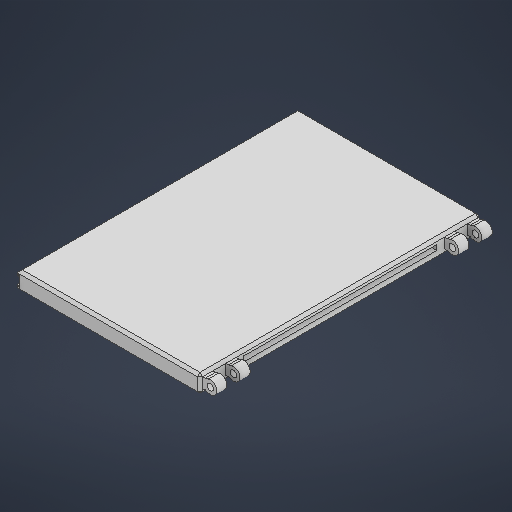
# Autodesk Inventor part: Деталь1
Saved by Autodesk Inventor 2025.1 (Build 291241000, 241)
## iProperties
Created: 2025-05-09
Part Number: Деталь1
Material: Типовые
Document SubType Name: Modeling
Designer: bogda
Density: 1 g/cm^3
Appearance: По умолчанию
Author: bogda
Autodesk Inventor part; units mm, degrees
ref_plane "YZ Plane" through (0, 0, 0) normal (1, 0, 0) x (0, 1, 0)
ref_plane "XZ Plane" through (0, 0, 0) normal (0, 1, 0) x (-1, 0, 0)
ref_plane "XY Plane" through (0, 0, 0) normal (0, 0, 1) x (1, 0, 0)
sketch "Эскиз1" plane through (0, 0, 0) normal (0, 1, 0) x (-1, 0, 0)
  line L0 (33.5, 52.5) -> (-33.5, 52.5)
  line L1 (-33.5, 52.5) -> (-33.5, -52.5)
  line L2 (-33.5, -52.5) -> (33.5, -52.5)
  line L3 (33.5, -52.5) -> (33.5, 52.5)
  line L4 (33.5, 52.5) -> (-33.5, -52.5) construction
  line L5 (-33.5, 52.5) -> (33.5, -52.5) construction
  line L6 (35.5, 54.5) -> (-35.5, 54.5)
  line L7 (-35.5, 54.5) -> (-35.5, -54.5)
  line L8 (-35.5, -54.5) -> (35.5, -54.5)
  line L9 (35.5, -54.5) -> (35.5, 54.5)
  point P0 (0, 0)
  dimension "d0" = 67
  dimension "d1" = 105
  dimension "d2" = 2
  constraints: 20 end point, 4 parallel, 2 midpoint, 2 perpendicular, 1 horizontal, 3 other
  measures "d0" distance of L2.end L1.end
  measures "d1" distance of L1.end L0.end
  measures "d2" distance between parallel lines of L3 L9
extrude "Выдавливание1" add sketch "Эскиз1" against normal blind 2 contours L3 L2 L1 L0 | L9 L8 L7 L6
extrude "Выдавливание2" add sketch "Эскиз1" against normal blind 6
sketch "Эскиз2" plane through (0, -6, 0) normal (0, -1, 0) x (1, 0, 0)
  line L0 (-33.5, -52.5) -> (-33.5, 52.5) projected
  line L1 (-33.5, -52.5) -> (-33.5, -49.5)
  line L2 (-33.5, -49.5) -> (33.5, -49.5)
  line L3 (33.5, 52.5) -> (33.5, -52.5) projected
  line L4 (33.5, -49.5) -> (26.5, -49.5)
  line L5 (26.5, -49.5) -> (26.5, 52.5)
  line L6 (-33.5, 52.5) -> (33.5, 52.5) projected
  line L7 (26.5, 52.5) -> (26.5, 49.5)
  line L8 (26.5, 49.5) -> (-33.5, 49.5)
  line L9 (-33.5, 49.5) -> (-30.5, 49.5)
  line L10 (-30.5, 49.5) -> (-30.5, -49.5)
  line L11 (33.5, -52.5) -> (-33.5, -52.5) projected
  line L12 (-33.5, -52.5) -> (33.5, -52.5)
  point P0 (0, 0)
  dimension "d7" = 3
  dimension "d8" = 7
  dimension "d9" = 3
  dimension "d10" = 3
  constraints: 18 end point, 8 point on line, 5 perpendicular
  measures "d7" distance of L0.start L1.end
  measures "d8" distance of L2.end L4.end
  measures "d9" distance of L5.end L7.end
  measures "d10" distance of L8.end L9.end
extrude "Выдавливание3" add sketch "Эскиз2" against normal blind 1 contours L0 L2 L3 L11 | L0 L8 L10 L2 | L0 L6 L5 L8 | L2 L5 L6 L3
sketch "Эскиз3" plane through (35.5, 0, 54.5) normal (1, 0, 0) x (0, 0, -1)
  line L0 (109, 0) -> (109, -6) projected
  line L1 (109, 0) -> (92, 0)
  line L2 (0, 0) -> (109, 0) projected
  line L3 (92, 0) -> (92, -2)
  line L4 (2, -5) -> (107, -5) projected
  line L5 (92, -2) -> (17, -2)
  line L6 (0, 0) -> (0, -6) projected
  line L7 (17, -2) -> (17, -4)
  line L8 (17, -4) -> (92, -4)
  line L9 (92, -4) -> (92, -2)
  line L10 (109, 0) -> (94, 0)
  line L11 (94, 0) -> (94, -6)
  line L12 (94, -6) -> (109, -6)
  line L13 (109, 0) -> (109, -6)
  line L14 (108, -5) -> (95, -5)
  line L15 (95, -5) -> (95, -1)
  line L16 (95, -1) -> (108, -1)
  line L17 (108, -1) -> (108, -5)
  line L18 (0, 0) -> (15, 0)
  line L19 (15, 0) -> (15, -6)
  line L20 (104, -6) -> (5, -6) projected
  line L21 (0, -6) -> (109, -6) projected
  line L22 (0, -6) -> (15, -6)
  line L23 (0, -6) -> (0, 0)
  line L24 (14, -5) -> (14, -1)
  line L25 (14, -1) -> (1, -1)
  line L26 (1, -1) -> (1, -5)
  line L27 (1, -5) -> (14, -5)
  line L28 (108, -5) -> (104, -5)
  line L29 (104, -5) -> (104, -1)
  line L30 (95, -5) -> (99, -5)
  line L31 (99, -5) -> (99, -1)
  line L32 (1, -5) -> (5, -5)
  line L33 (5, -5) -> (5, -1)
  line L34 (14, -5) -> (10, -5)
  line L35 (10, -5) -> (10, -1)
  point P0 (54.5, 0)
  point P1 (5, -5)
  point P2 (10, -5)
  point P3 (14, -5)
  dimension "d13" = 17
  dimension "d14" = 2
  dimension "d15" = 75
  dimension "d16" = 2
  dimension "d17" = 15
  dimension "d18" = 1
  dimension "d19" = 15
  dimension "d20" = 1
  dimension "d21" = 4
  dimension "d22" = 4
  dimension "d23" = 4
  dimension "d24" = 4
  constraints: 60 end point, 16 perpendicular, 12 point on line, 2 collinear, 6 other
  measures "d13" distance of L0.start L1.end
  measures "d14" distance of L1.end L3.end
  measures "d15" distance of L3.end L5.end
  measures "d16" distance of L5.end L7.end
  measures "d17" distance of L0.start L10.end
  measures "d18" distance between parallel lines of L12 L14
  measures "d19" distance of L2.start L18.end
  measures "d20" distance between parallel lines of L22 L27
  measures "d21" distance of L14.start L28.end
  measures "d22" distance of L14.end L30.end
  measures "d23" distance of L26.end L32.end
  measures "d24" distance of L24.start L34.end
extrude "Выдавливание4" cut sketch "Эскиз3" against normal blind 3 contours L9 L8 L7 L5
extrude "Выдавливание5" add sketch "Эскиз3" along normal blind 1 contours L27 L26 L25 L33 L4 | L35 L25 L24 L4 | L15 L16 L31 L4 | L29 L16 L17 L14 L4
sketch "Эскиз4" plane through (35.5, -5, -53.5) normal (0, 0, -1) x (-1, 0, 0)
  line L0 (-1, 4) -> (-1, 0) projected
  line L1 (-1, 0) -> (-1, 2)
  line L2 (-1, 2) -> (-3, 2)
  circle A0 centre (-3, 2) radius 2.5
  line L3 (-1, 0) -> (-2.2643, -0.3893)
  line L4 (-1, 4) -> (-2.2643, 4.3893)
  circle A1 centre (-3, 2) radius 1.25
  point P0 (35.5, 5)
  dimension "d29" = 2
  dimension "d30" = 2
  dimension "d31" = 5
  dimension "d32" = 2.5
  constraints: 8 end point, 2 centre point, 2 coincident, 2 point on circle, 2 tangent, 1 midpoint, 1 perpendicular
  measures "d29" distance of L0.end L1.end
  measures "d30" distance of L1.end L2.end
  measures "d31" diameter of A0
  measures "d32" diameter of A1
extrude "Выдавливание6" add sketch "Эскиз4" against normal blind 107 contours L0 A0 L4 | L0 A0 | A0 L0 L3 picked at (-1.2977, 1.3064)
sketch "Эскиз5" plane through (35.5, -5, -49.5) normal (0, 0, 1) x (1, 0, 0)
  line L0 (1, 0) -> (1, 4) projected
  line L1 (1, 0) -> (1, -1.4659)
  line L2 (1, -1.4659) -> (6.5669, -1.4659)
  line L3 (6.5669, -1.4659) -> (6.5669, 5)
  line L4 (6.5669, 5) -> (1, 5)
  line L5 (1, 5) -> (1, 4)
  line L6 (1, 4) -> (1, 0)
  point P0 (-35.5, 5)
  constraints: 12 end point, 4 perpendicular, 1 collinear, 1 point on line, 1 vertical
extrude "Выдавливание7" cut sketch "Эскиз5" along normal blind 5
sketch "Эскиз6" plane through (35.5, -5, -40.5) normal (0, 0, 1) x (1, 0, 0)
  line L0 (1, 0) -> (1, 4) projected
  line L1 (1, 0) -> (1, -1.1885)
  line L2 (1, -1.1885) -> (6.8207, -1.1885)
  line L3 (6.8207, -1.1885) -> (6.8207, 5)
  line L4 (6.8207, 5) -> (1, 5)
  line L5 (1, 5) -> (1, 4)
  line L6 (1, 4) -> (1, 0)
  point P0 (-35.5, 5)
  constraints: 12 end point, 4 perpendicular, 1 collinear, 1 point on line, 1 vertical
extrude "Выдавливание8" cut sketch "Эскиз6" along normal blind 81
sketch "Эскиз7" plane through (35.5, -5, 44.5) normal (0, 0, 1) x (1, 0, 0)
  line L0 (1, 0) -> (1, 4) projected
  line L1 (1, 4) -> (1, 5.6826)
  line L2 (1, 5.6826) -> (6.1559, 5.6826)
  line L3 (6.1559, 5.6826) -> (6.1559, -0.9821)
  line L4 (6.1559, -0.9821) -> (1, -0.9821)
  line L5 (1, -0.9821) -> (1, 0)
  line L6 (1, 0) -> (1, 4)
  point P0 (-35.5, 5)
  constraints: 12 end point, 3 perpendicular, 2 collinear, 1 point on line, 1 vertical
extrude "Выдавливание9" cut sketch "Эскиз7" along normal blind 5
sketch "Эскиз8" plane through (-35.5, 0, -54.5) normal (-1, 0, 0) x (0, 0, 1)
  line L0 (1, -5) -> (5, -5) projected
  line L1 (5, -1) -> (1, -1) projected
  line L2 (0, 0) -> (0, -6) projected
  line L3 (0, -5) -> (2, -5)
  line L4 (2, -5) -> (2, -2)
  line L5 (0, 0) -> (109, 0) projected
  line L6 (107, -2) -> (107, -5) projected
  line L7 (2, -2) -> (107, -2)
  line L8 (107, -2) -> (107, -5)
  line L9 (107, -5) -> (2, -5)
  point P0 (54.5, 0)
  dimension "d41" = 2
  dimension "d42" = 3
  constraints: 10 end point, 2 collinear, 2 point on line, 1 perpendicular
  measures "d41" distance of L3.start L3.end
  measures "d42" distance of L3.end L4.end
extrude "Выдавливание10" cut sketch "Эскиз8" against normal blind 5
sketch "Эскиз9" plane through (-35.5, 0, 54.5) normal (0, 0, 1) x (1, 0, 0)
  line L0 (0, 0) -> (0, -2)
  line L1 (0, 0) -> (0, -6) projected
  line L2 (0, -2) -> (0.5, -2)
  line L3 (0.5, -2) -> (0.5, 0)
  line L4 (0.5, 0) -> (1, 0)
  line L5 (1, 0) -> (1, -5)
  line L6 (1, -5) -> (1, -5.5)
  line L7 (1, -5.5) -> (0.5, -5.5)
  line L8 (0.5, -5.5) -> (0.5, -5)
  line L9 (0.5, -5) -> (0, -5)
  line L10 (0, -5) -> (0, -2)
  line L11 (0.5, 0) -> (0.5, -1)
  line L12 (0.5, -1) -> (1, -1)
  point P0 (35.5, 0)
  dimension "d45" = 2
  dimension "d46" = 0.5
  dimension "d47" = 0.5
  dimension "d48" = 5
  dimension "d49" = 0.5
  dimension "d50" = 1
  constraints: 24 end point, 8 perpendicular, 6 point on line, 1 midpoint
  measures "d45" distance of L0.start L0.end
  measures "d46" distance of L0.end L2.end
  measures "d47" distance of L3.end L4.end
  measures "d48" distance of L4.end L5.end
  measures "d49" distance of L5.end L6.end
  measures "d50" distance of L3.end L11.end
extrude "Выдавливание11" cut sketch "Эскиз9" against normal blind 110 contours L2 L3 L12 L5 L6 L7 L8 L9 L1
sketch "Эскиз10" plane through (0, -6, 0) normal (0, -1, 0) x (1, 0, 0)
  line L0 (35.5, 54.5) -> (-35.5, 54.5) projected
  line L1 (-35.5, 54.5) -> (-35.5, 52.5)
  line L2 (-35.5, 52.5) -> (35.5, 52.5)
  line L3 (35.5, -54.5) -> (35.5, 54.5) projected
  line L4 (35.5, 52.5) -> (33.5, 52.5)
  line L5 (33.5, 52.5) -> (33.5, -54.5)
  line L6 (-35.5, -54.5) -> (35.5, -54.5) projected
  line L7 (33.5, -54.5) -> (33.5, -52.5)
  line L8 (33.5, -52.5) -> (-35.5, -52.5)
  line L9 (-35.5, -52.5) -> (-33.5, -52.5)
  line L10 (-33.5, -52.5) -> (-33.5, 52.5)
  line L11 (-35.5, 52.5) -> (-35.5, -52.5)
  line L12 (-35.5, -52.5) -> (-35.5, -54.5)
  line L13 (28.1404, -7.8899) -> (28.1404, 8.4295) construction
  line L14 (28.1404, 8.4295) -> (34.5634, 8.4295) construction
  line L15 (34.5634, 8.4295) -> (34.5634, -7.8899) construction
  line L16 (34.5634, -7.8899) -> (28.1404, -7.8899) construction
  spline S0 degree 2 poles (29.8027, -5.1778) (30.2201, -5.1778) (30.892, -5.5162) (31.0797, -5.8002) knots 0 0 0 1 2 2 2
  spline S1 degree 2 poles (31.0797, -5.8002) (31.2254, -6.0324) (31.3242, -6.5091) (31.3242, -6.8796) knots 0 0 0 1 2 2 2
  line L17 (31.3242, -6.8796) -> (31.3242, -7.5811)
  line L18 (31.3242, -7.5811) -> (28.2762, -7.5811)
  line L19 (28.2762, -7.5811) -> (28.2762, -6.887)
  spline S2 degree 2 poles (28.2762, -6.887) (28.2762, -6.4573) (28.4047, -5.9682) (28.5183, -5.7953) knots 0 0 0 1 2 2 2
  spline S3 degree 2 poles (28.5183, -5.7953) (28.7134, -5.5014) (29.3581, -5.1778) (29.8027, -5.1778) knots 0 0 0 1 2 2 2
  spline S4 degree 2 poles (29.7978, -5.6002) (29.447, -5.6002) (28.9506, -5.8323) (28.8098, -6.0621) knots 0 0 0 1 2 2 2
  spline S5 degree 2 poles (28.8098, -6.0621) (28.7134, -6.2251) (28.627, -6.5931) (28.627, -6.8673) knots 0 0 0 1 2 2 2
  line L20 (28.627, -6.8673) -> (28.627, -7.176)
  line L21 (28.627, -7.176) -> (30.9735, -7.176)
  line L22 (30.9735, -7.176) -> (30.9735, -6.8673)
  spline S6 degree 2 poles (30.9735, -6.8673) (30.9735, -6.5981) (30.887, -6.1905) (30.771, -6.025) knots 0 0 0 1 2 2 2
  spline S7 degree 2 poles (30.771, -6.025) (30.6277, -5.8126) (30.1535, -5.6002) (29.7978, -5.6002) knots 0 0 0 1 2 2 2
  line L23 (31.3242, -2.9894) -> (31.3242, -3.3747)
  line L24 (31.3242, -3.3747) -> (31.0723, -3.3747)
  spline S8 degree 2 poles (31.0723, -3.3747) (31.2279, -3.5525) (31.3885, -3.8712) (31.3885, -4.0688) knots 0 0 0 1 2 2 2
  spline S9 degree 2 poles (31.3885, -4.0688) (31.3885, -4.217) (31.2897, -4.4812) (31.1835, -4.5776) knots 0 0 0 1 2 2 2
  spline S10 degree 2 poles (31.1835, -4.5776) (31.0772, -4.6764) (30.7537, -4.7851) (30.5215, -4.7851) knots 0 0 0 1 2 2 2
  line L25 (30.5215, -4.7851) -> (29.037, -4.7851)
  line L26 (29.037, -4.7851) -> (29.037, -4.3997)
  line L27 (29.037, -4.3997) -> (30.3412, -4.3997)
  spline S11 degree 2 poles (30.3412, -4.3997) (30.524, -4.3997) (30.7635, -4.3726) (30.8525, -4.3256) knots 0 0 0 1 2 2 2
  spline S12 degree 2 poles (30.8525, -4.3256) (30.9414, -4.2787) (31.0229, -4.1182) (31.0229, -3.9675) knots 0 0 0 1 2 2 2
  spline S13 degree 2 poles (31.0229, -3.9675) (31.0229, -3.8267) (30.8623, -3.5081) (30.7463, -3.3747) knots 0 0 0 1 2 2 2
  line L28 (30.7463, -3.3747) -> (29.037, -3.3747)
  line L29 (29.037, -3.3747) -> (29.037, -2.9894)
  line L30 (29.037, -2.9894) -> (31.3242, -2.9894)
  spline S14 degree 2 poles (31.3761, -1.5222) (31.3761, -1.7593) (31.2304, -2.152) (31.0822, -2.2928) knots 0 0 0 1 2 2 2
  spline S15 degree 2 poles (31.0822, -2.2928) (30.9364, -2.4336) (30.4869, -2.5892) (30.1856, -2.5892) knots 0 0 0 1 2 2 2
  spline S16 degree 2 poles (30.1856, -2.5892) (29.8842, -2.5892) (29.4446, -2.4287) (29.2964, -2.2928) knots 0 0 0 1 2 2 2
  spline S17 degree 2 poles (29.2964, -2.2928) (29.1457, -2.157) (28.9851, -1.7543) (28.9851, -1.5222) knots 0 0 0 1 2 2 2
  spline S18 degree 2 poles (28.9851, -1.5222) (28.9851, -1.3344) (29.0913, -0.9837) (29.1605, -0.8479) knots 0 0 0 1 2 2 2
  line L31 (29.1605, -0.8479) -> (29.5928, -0.8479)
  line L32 (29.5928, -0.8479) -> (29.5928, -0.8701)
  spline S19 degree 2 poles (29.5928, -0.8701) (29.5582, -0.9121) (29.4693, -1.0405) (29.4223, -1.1319) knots 0 0 0 1 2 2 2
  spline S20 degree 2 poles (29.4223, -1.1319) (29.3828, -1.2134) (29.3211, -1.4308) (29.3211, -1.5296) knots 0 0 0 1 2 2 2
  spline S21 degree 2 poles (29.3211, -1.5296) (29.3211, -1.8284) (29.7731, -2.1915) (30.1856, -2.1915) knots 0 0 0 1 2 2 2
  spline S22 degree 2 poles (30.1856, -2.1915) (30.5882, -2.1915) (31.0402, -1.8408) (31.0402, -1.5296) knots 0 0 0 1 2 2 2
  spline S23 degree 2 poles (31.0402, -1.5296) (31.0402, -1.3419) (30.8846, -1.001) (30.7635, -0.8701) knots 0 0 0 1 2 2 2
  line L33 (30.7635, -0.8701) -> (30.7635, -0.8479)
  line L34 (30.7635, -0.8479) -> (31.1958, -0.8479)
  spline S24 degree 2 poles (31.1958, -0.8479) (31.223, -0.9047) (31.2995, -1.0776) (31.3168, -1.1467) knots 0 0 0 1 2 2 2
  spline S25 degree 2 poles (31.3168, -1.1467) (31.3465, -1.2455) (31.3761, -1.4011) (31.3761, -1.5222) knots 0 0 0 1 2 2 2
  line L35 (31.3242, 1.3974) -> (31.3242, 0.891)
  line L36 (31.3242, 0.891) -> (30.2201, 0.0414)
  line L37 (30.2201, 0.0414) -> (30.3683, -0.1118)
  line L38 (30.3683, -0.1118) -> (31.3242, -0.1118)
  line L39 (31.3242, -0.1118) -> (31.3242, -0.4971)
  line L40 (31.3242, -0.4971) -> (28.1404, -0.4971)
  line L41 (28.1404, -0.4971) -> (28.1404, -0.1118)
  line L42 (28.1404, -0.1118) -> (30.0028, -0.1118)
  line L43 (30.0028, -0.1118) -> (29.037, 0.7922)
  line L44 (29.037, 0.7922) -> (29.037, 1.2714)
  line L45 (29.037, 1.2714) -> (29.9929, 0.3328)
  line L46 (29.9929, 0.3328) -> (31.3242, 1.3974)
  spline S26 degree 2 poles (30.3881, 3.6871) (30.6153, 3.6871) (30.9636, 3.5142) (31.0772, 3.3709) knots 0 0 0 1 2 2 2
  spline S27 degree 2 poles (31.0772, 3.3709) (31.2106, 3.198) (31.3242, 2.8053) (31.3242, 2.4941) knots 0 0 0 1 2 2 2
  line L47 (31.3242, 2.4941) -> (31.3242, 1.6197)
  line L48 (31.3242, 1.6197) -> (28.2762, 1.6197)
  line L49 (28.2762, 1.6197) -> (28.2762, 2.4274)
  spline S28 degree 2 poles (28.2762, 2.4274) (28.2762, 2.7534) (28.3182, 3.0795) (28.3997, 3.2277) knots 0 0 0 1 2 2 2
  spline S29 degree 2 poles (28.3997, 3.2277) (28.4862, 3.3932) (28.7702, 3.5438) (28.9629, 3.5438) knots 0 0 0 1 2 2 2
  spline S30 degree 2 poles (28.9629, 3.5438) (29.1778, 3.5438) (29.5187, 3.3166) (29.615, 3.1165) knots 0 0 0 1 2 2 2
  line L50 (29.615, 3.1165) -> (29.6298, 3.1165)
  spline S31 degree 2 poles (29.6298, 3.1165) (29.7039, 3.3882) (30.0966, 3.6871) (30.3881, 3.6871) knots 0 0 0 1 2 2 2
  spline S32 degree 2 poles (30.4054, 3.2647) (30.2325, 3.2647) (30.0102, 3.1659) (29.9312, 3.0177) knots 0 0 0 1 2 2 2
  spline S33 degree 2 poles (29.9312, 3.0177) (29.8818, 2.9214) (29.8521, 2.6942) (29.8521, 2.4842) knots 0 0 0 1 2 2 2
  line L51 (29.8521, 2.4842) -> (29.8521, 2.0248)
  line L52 (29.8521, 2.0248) -> (30.9784, 2.0248)
  line L53 (30.9784, 2.0248) -> (30.9784, 2.3533)
  spline S34 degree 2 poles (30.9784, 2.3533) (30.9784, 2.6201) (30.929, 2.9263) (30.85, 3.0449) knots 0 0 0 1 2 2 2
  spline S35 degree 2 poles (30.85, 3.0449) (30.7685, 3.1585) (30.5659, 3.2647) (30.4054, 3.2647) knots 0 0 0 1 2 2 2
  spline S36 degree 2 poles (29.0197, 3.1215) (28.911, 3.1215) (28.748, 3.0474) (28.7011, 2.9659) knots 0 0 0 1 2 2 2
  spline S37 degree 2 poles (28.7011, 2.9659) (28.6467, 2.8671) (28.622, 2.6275) (28.622, 2.4126) knots 0 0 0 1 2 2 2
  line L54 (28.622, 2.4126) -> (28.622, 2.0248)
  line L55 (28.622, 2.0248) -> (29.5137, 2.0248)
  line L56 (29.5137, 2.0248) -> (29.5137, 2.4842)
  spline S38 degree 2 poles (29.5137, 2.4842) (29.5137, 2.6744) (29.4742, 2.8547) (29.4124, 2.951) knots 0 0 0 1 2 2 2
  spline S39 degree 2 poles (29.4124, 2.951) (29.3532, 3.0449) (29.163, 3.1215) (29.0197, 3.1215) knots 0 0 0 1 2 2 2
  line L57 (31.3242, 4.4528) -> (31.3242, 4.0675)
  line L58 (31.3242, 4.0675) -> (29.037, 4.0675)
  line L59 (29.037, 4.0675) -> (29.037, 4.4528)
  line L60 (29.037, 4.4528) -> (31.3242, 4.4528)
  line L61 (28.6566, 4.48) -> (28.6566, 4.0428)
  line L62 (28.6566, 4.0428) -> (28.2565, 4.0428)
  line L63 (28.2565, 4.0428) -> (28.2565, 4.48)
  line L64 (28.2565, 4.48) -> (28.6566, 4.48)
  spline S40 degree 2 poles (31.3687, 5.71) (31.3687, 5.3963) (31.0105, 5.0431) (30.6228, 5.0431) knots 0 0 0 1 2 2 2
  line L65 (30.6228, 5.0431) -> (29.3556, 5.0431)
  line L66 (29.3556, 5.0431) -> (29.3556, 4.7838)
  line L67 (29.3556, 4.7838) -> (29.037, 4.7838)
  line L68 (29.037, 4.7838) -> (29.037, 5.0431)
  line L69 (29.037, 5.0431) -> (28.38, 5.0431)
  line L70 (28.38, 5.0431) -> (28.38, 5.4285)
  line L71 (28.38, 5.4285) -> (29.037, 5.4285)
  line L72 (29.037, 5.4285) -> (29.037, 6.1374)
  line L73 (29.037, 6.1374) -> (29.3556, 6.1374)
  line L74 (29.3556, 6.1374) -> (29.3556, 5.4285)
  line L75 (29.3556, 5.4285) -> (30.4449, 5.4285)
  spline S41 degree 2 poles (30.4449, 5.4285) (30.6178, 5.4285) (30.808, 5.4408) (30.8895, 5.4828) knots 0 0 0 1 2 2 2
  spline S42 degree 2 poles (30.8895, 5.4828) (30.9611, 5.5174) (31.0328, 5.673) (31.0328, 5.8064) knots 0 0 0 1 2 2 2
  spline S43 degree 2 poles (31.0328, 5.8064) (31.0328, 5.9002) (30.976, 6.0756) (30.9587, 6.1151) knots 0 0 0 1 2 2 2
  line L76 (30.9587, 6.1151) -> (30.9587, 6.1374)
  line L77 (30.9587, 6.1374) -> (31.3045, 6.1374)
  spline S44 degree 2 poles (31.3045, 6.1374) (31.3341, 6.0287) (31.3687, 5.8064) (31.3687, 5.71) knots 0 0 0 1 2 2 2
  line L78 (31.3242, 8.0911) -> (31.3242, 6.6042)
  line L79 (31.3242, 6.6042) -> (31.013, 6.6042)
  line L80 (31.013, 6.6042) -> (31.013, 7.1575)
  line L81 (31.013, 7.1575) -> (28.9703, 7.1575)
  line L82 (28.9703, 7.1575) -> (28.9703, 6.6042)
  line L83 (28.9703, 6.6042) -> (28.6912, 6.6042)
  spline S45 degree 2 poles (28.6912, 6.6042) (28.6912, 6.9179) (28.5134, 7.2143) (28.2664, 7.234) knots 0 0 0 1 2 2 2
  line L84 (28.2664, 7.234) -> (28.2664, 7.5502)
  line L85 (28.2664, 7.5502) -> (31.013, 7.5502)
  line L86 (31.013, 7.5502) -> (31.013, 8.0911)
  line L87 (31.013, 8.0911) -> (31.3242, 8.0911)
  point P0 (0, 0)
  dimension "d0" = 67
  dimension "d1" = 105
  dimension "d2" = 2
  dimension "d53" = 2
  dimension "d54" = 2
  dimension "d55" = 2
  dimension "d56" = 2
  constraints: 20 end point, 7 point on line, 4 perpendicular, 2 vertical, 1 parallel, 2 other
  measures "d53" distance of L0.end L1.end
  measures "d54" distance of L2.end L4.end
  measures "d55" distance of L5.end L7.end
  measures "d56" distance of L8.end L9.end
extrude "Выдавливание12" add sketch "Эскиз10" along normal blind 1 contours L3 L2 L1 L0 | L3 L6 L5 L2 | L2 L10 L8 L11 | L8 L5 L6 L12
extrude "Выдавливание13" add sketch "Эскиз10" along normal blind 0.5 contours S0 S1 L17 L18 L19 S2 S3 | L23 L24 S8 S9 S10 L25 L26 L27 S11 S12 S13 L28 L29 L30 | S14 S15 S16 S17 S18 L31 L32 S19 S20 S21 S22 S23 L33 L34 S24 S25 | L35 L36 L37 L38 L39 L40 L41 L42 L43 L44 L45 L46 | S26 S27 L47 L48 L49 S28 S29 S30 L50 S31 | L57 L58 L59 L60 | L61 L62 L63 L64 | S40 L65 L66 L67 L68 L69 L70 L71 L72 L73 L74 L75 S41 S42 S43 L76 L77 S44 | L78 L79 L80 L81 L82 L83 S45 L84 L85 L86 L87
chamfer "Фаска1" distance 1 angle 45 14 edges at (-35.5, 0, 0) (0, 0, -54.5) (35.5, 0, 0) (0, 0, 54.5) (35.5, -3.5, 54.5) (35.5, -3.5, -54.5) (0, -7, -54.5) (-35.5, -7, 0) (35.5, -7, 0) (0, -7, 54.5) (0, -6, 52.5) (-33.5, -6, 0) (0, -6, -52.5) (33.5, -6, 0)
chamfer "Фаска2" distance 1 angle 45 2 edges at (-34.5, -3.5, -52.5) (-34.5, -3.5, 52.5)
